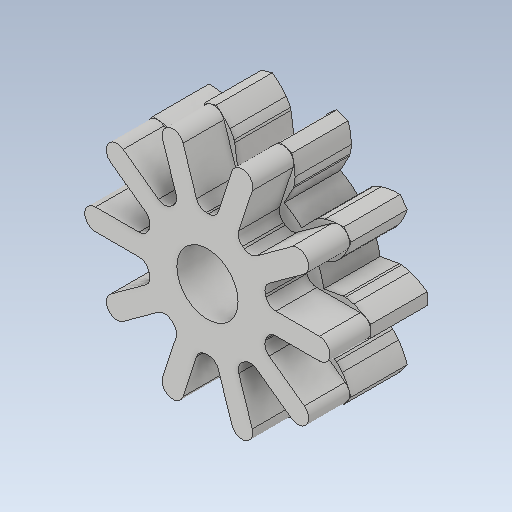
# Autodesk Inventor part: m2z10はめあい
Saved by Autodesk Inventor 2020 (Build 240168000, 168)
## iProperties
Created: 2019-05-28
Part Number: m2z10はめあい
Material: 一般
Document SubType Name: Modeling
Designer: hamaa
Density: 1 g/cm^3
Appearance: 既定
Mass: 2.32031 g
Surface Area: 20.1753 cm^2
Volume: 2.32031 cm^3
Author: hamaa
Autodesk Inventor part; units mm, degrees
ref_plane "YZ Plane" through (0, 0, 0) normal (1, 0, 0) x (0, 1, 0)
ref_plane "XZ Plane" through (0, 0, 0) normal (0, 1, 0) x (-1, 0, 0)
ref_plane "XY Plane" through (0, 0, 0) normal (0, 0, 1) x (1, 0, 0)
sketch "スケッチ1" plane through (0, 0, 0) normal (0, 0, 1) x (1, 0, 0)
  arc A0 (149.895, 114.5174) -> (149.8316, 114.302) centre (151.0075, 114.073) ccw
  arc A1 (150.3048, 115.256) -> (149.895, 114.5174) centre (153.0017, 113.2765) ccw
  arc A2 (151.645, 116.5804) -> (150.3048, 115.256) centre (155.1281, 111.7157) ccw
  arc A3 (144.0343, 113.5196) -> (144.1097, 113.3081) centre (145.1956, 113.8141) ccw
  arc A4 (143.9318, 114.3581) -> (144.0343, 113.5196) centre (147.2771, 114.3418) ccw
  arc A5 (144.2375, 116.2174) -> (143.9318, 114.3581) centre (149.9148, 114.329) ccw
  arc A6 (139.8794, 109.2677) -> (140.0647, 109.1408) centre (140.6459, 110.1884) ccw
  arc A7 (139.3036, 109.8857) -> (139.8794, 109.2677) centre (142.0196, 111.8388) ccw
  arc A8 (138.4581, 111.5696) -> (139.3036, 109.8857) centre (144.1611, 113.3789) ccw
  arc A9 (139.0173, 103.3856) -> (139.2417, 103.3918) centre (139.0961, 104.581) ccw
  arc A10 (138.1882, 103.5471) -> (139.0173, 103.3856) centre (139.2374, 106.7236) ccw
  arc A11 (136.5144, 104.4124) -> (138.1882, 103.5471) centre (140.0647, 109.2283) ccw
  arc A12 (141.7772, 98.1201) -> (141.9551, 98.2571) centre (141.1383, 99.1335) ccw
  arc A13 (141.0115, 97.7634) -> (141.7772, 98.1201) centre (139.9932, 100.95) ccw
  arc A14 (139.1487, 97.4797) -> (141.0115, 97.7634) centre (139.1903, 103.4626) ccw
  arc A15 (147.105, 95.4824) -> (147.1684, 95.6978) centre (145.9925, 95.9268) ccw
  arc A16 (146.6952, 94.7438) -> (147.105, 95.4824) centre (143.9983, 96.7233) ccw
  arc A17 (145.355, 93.4194) -> (146.6952, 94.7438) centre (141.8719, 98.2841) ccw
  arc A18 (152.9656, 96.4802) -> (152.8903, 96.6917) centre (151.8044, 96.1857) ccw
  arc A19 (153.0682, 95.6417) -> (152.9656, 96.4802) centre (149.7229, 95.658) ccw
  arc A20 (152.7625, 93.7824) -> (153.0682, 95.6417) centre (147.0852, 95.6708) ccw
  arc A21 (157.1206, 100.7321) -> (156.9353, 100.859) centre (156.3541, 99.8114) ccw
  arc A22 (157.6964, 100.1141) -> (157.1206, 100.7321) centre (154.9804, 98.161) ccw
  arc A23 (158.5419, 98.4302) -> (157.6964, 100.1141) centre (152.8389, 96.6209) ccw
  arc A24 (157.9827, 106.6143) -> (157.7583, 106.608) centre (157.9039, 105.4188) ccw
  arc A25 (158.8118, 106.4527) -> (157.9827, 106.6143) centre (157.7626, 103.2762) ccw
  arc A26 (160.4856, 105.5874) -> (158.8118, 106.4527) centre (156.9353, 100.7715) ccw
  arc A27 (155.2228, 111.8797) -> (155.0449, 111.7427) centre (155.8617, 110.8663) ccw
  arc A28 (155.9885, 112.2364) -> (155.2228, 111.8797) centre (157.0068, 109.0498) ccw
  arc A29 (157.8512, 112.5201) -> (155.9885, 112.2364) centre (157.8097, 106.5372) ccw
  arc A30 (147.1684, 114.302) -> (147.105, 114.5174) centre (145.9925, 114.073) ccw
  arc A31 (147.105, 114.5174) -> (146.6952, 115.256) centre (143.9983, 113.2765) ccw
  arc A32 (146.6952, 115.256) -> (145.355, 116.5804) centre (141.8719, 111.7157) ccw
  arc A33 (141.9551, 111.7427) -> (141.7772, 111.8797) centre (141.1383, 110.8663) ccw
  arc A34 (141.7772, 111.8797) -> (141.0115, 112.2364) centre (139.9932, 109.0498) ccw
  arc A35 (141.0115, 112.2364) -> (139.1487, 112.5201) centre (139.1903, 106.5372) ccw
  arc A36 (139.2417, 106.608) -> (139.0173, 106.6143) centre (139.0961, 105.4188) ccw
  arc A37 (139.0173, 106.6143) -> (138.1882, 106.4527) centre (139.2374, 103.2762) ccw
  arc A38 (138.1882, 106.4527) -> (136.5144, 105.5874) centre (140.0647, 100.7715) ccw
  arc A39 (140.0647, 100.859) -> (139.8794, 100.7321) centre (140.6459, 99.8114) ccw
  arc A40 (139.8794, 100.7321) -> (139.3036, 100.1141) centre (142.0196, 98.161) ccw
  arc A41 (139.3036, 100.1141) -> (138.4581, 98.4302) centre (144.1611, 96.6209) ccw
  arc A42 (144.1097, 96.6917) -> (144.0343, 96.4802) centre (145.1956, 96.1857) ccw
  arc A43 (144.0343, 96.4802) -> (143.9318, 95.6417) centre (147.2771, 95.658) ccw
  arc A44 (143.9318, 95.6417) -> (144.2375, 93.7824) centre (149.9148, 95.6708) ccw
  arc A45 (149.8316, 95.6978) -> (149.895, 95.4824) centre (151.0075, 95.9268) ccw
  arc A46 (149.895, 95.4824) -> (150.3048, 94.7438) centre (153.0017, 96.7233) ccw
  arc A47 (150.3048, 94.7438) -> (151.645, 93.4194) centre (155.1281, 98.2841) ccw
  arc A48 (155.0449, 98.2571) -> (155.2228, 98.1201) centre (155.8617, 99.1335) ccw
  arc A49 (155.2228, 98.1201) -> (155.9885, 97.7634) centre (157.0068, 100.95) ccw
  arc A50 (155.9885, 97.7634) -> (157.8512, 97.4797) centre (157.8097, 103.4626) ccw
  arc A51 (157.7583, 103.3918) -> (157.9827, 103.3856) centre (157.9039, 104.581) ccw
  arc A52 (157.9827, 103.3856) -> (158.8118, 103.5471) centre (157.7626, 106.7236) ccw
  arc A53 (158.8118, 103.5471) -> (160.4856, 104.4124) centre (156.9353, 109.2283) ccw
  arc A54 (156.9353, 109.1408) -> (157.1206, 109.2677) centre (156.3541, 110.1884) ccw
  arc A55 (157.1206, 109.2677) -> (157.6964, 109.8857) centre (154.9804, 111.8388) ccw
  arc A56 (157.6964, 109.8857) -> (158.5419, 111.5696) centre (152.8389, 113.3789) ccw
  arc A57 (152.8903, 113.3081) -> (152.9656, 113.5196) centre (151.8044, 113.8141) ccw
  arc A58 (152.9656, 113.5196) -> (153.0682, 114.3581) centre (149.7229, 114.3418) ccw
  arc A59 (153.0682, 114.3581) -> (152.7625, 116.2174) centre (147.0852, 114.329) ccw
  arc A60 (149.5628, 112.4242) -> (147.4372, 112.4242) centre (148.5, 104.9999) ccw
  arc A61 (144.9959, 111.631) -> (143.2763, 110.3816) centre (148.5, 104.9999) ccw
  arc A62 (141.7675, 108.3049) -> (141.1106, 106.2833) centre (148.5, 104.9999) ccw
  arc A63 (141.1106, 103.7165) -> (141.7675, 101.6949) centre (148.5, 104.9999) ccw
  arc A64 (143.2763, 99.6182) -> (144.9959, 98.3688) centre (148.5, 104.9999) ccw
  arc A65 (147.4372, 97.5756) -> (149.5628, 97.5756) centre (148.5, 104.9999) ccw
  arc A66 (152.0041, 98.3688) -> (153.7237, 99.6182) centre (148.5, 104.9999) ccw
  arc A67 (155.2325, 101.6949) -> (155.8894, 103.7165) centre (148.5, 104.9999) ccw
  arc A68 (155.8894, 106.2833) -> (155.2325, 108.3049) centre (148.5, 104.9999) ccw
  arc A69 (153.7237, 110.3816) -> (152.0041, 111.631) centre (148.5, 104.9999) ccw
  arc A70 (145.355, 116.5804) -> (144.2375, 116.2174) centre (148.5, 104.9999) ccw
  arc A71 (139.1487, 112.5201) -> (138.4581, 111.5696) centre (148.5, 104.9999) ccw
  arc A72 (136.5144, 105.5874) -> (136.5144, 104.4124) centre (148.5, 104.9999) ccw
  arc A73 (138.4581, 98.4302) -> (139.1487, 97.4797) centre (148.5, 104.9999) ccw
  arc A74 (144.2375, 93.7824) -> (145.355, 93.4194) centre (148.5, 104.9999) ccw
  arc A75 (151.645, 93.4194) -> (152.7625, 93.7824) centre (148.5, 104.9999) ccw
  arc A76 (157.8512, 97.4797) -> (158.5419, 98.4302) centre (148.5, 104.9999) ccw
  arc A77 (160.4856, 104.4124) -> (160.4856, 105.5874) centre (148.5, 104.9999) ccw
  arc A78 (158.5419, 111.5696) -> (157.8512, 112.5201) centre (148.5, 104.9999) ccw
  arc A79 (152.7625, 116.2174) -> (151.645, 116.5804) centre (148.5, 104.9999) ccw
  line L0 (149.5628, 112.4242) -> (149.8316, 114.302)
  line L1 (144.9959, 111.631) -> (144.1097, 113.3081)
  line L2 (141.7675, 108.3049) -> (140.0647, 109.1408)
  line L3 (141.1106, 103.7165) -> (139.2417, 103.3918)
  line L4 (143.2763, 99.6182) -> (141.9551, 98.2571)
  line L5 (147.4372, 97.5756) -> (147.1684, 95.6978)
  line L6 (152.0041, 98.3688) -> (152.8903, 96.6917)
  line L7 (155.2325, 101.6949) -> (156.9353, 100.859)
  line L8 (155.8894, 106.2833) -> (157.7583, 106.608)
  line L9 (153.7237, 110.3816) -> (155.0449, 111.7427)
  line L10 (147.4372, 112.4242) -> (147.1684, 114.302)
  line L11 (143.2763, 110.3816) -> (141.9551, 111.7427)
  line L12 (141.1106, 106.2833) -> (139.2417, 106.608)
  line L13 (141.7675, 101.6949) -> (140.0647, 100.859)
  line L14 (144.9959, 98.3688) -> (144.1097, 96.6917)
  line L15 (149.5628, 97.5756) -> (149.8316, 95.6978)
  line L16 (153.7237, 99.6182) -> (155.0449, 98.2571)
  line L17 (155.8894, 103.7165) -> (157.7583, 103.3918)
  line L18 (155.2325, 108.3049) -> (156.9353, 109.1408)
  line L19 (152.0041, 111.631) -> (152.8903, 113.3081)
  line L20 (134.5, 105) -> (162.5, 105)
  line L21 (148.5, 91) -> (148.5, 119)
  line L22 (180.5, 116.9999) -> (250.5, 116.9999)
  line L23 (180.5, 108.9999) -> (250.5, 108.9999)
  line L24 (180.5, 100.9999) -> (250.5, 100.9999)
  line L25 (180.5, 92.9999) -> (250.5, 92.9999)
  line L26 (180.5, 84.9999) -> (250.5, 84.9999)
  line L27 (180.5, 76.9999) -> (250.5, 76.9999)
  line L28 (180.5, 68.9999) -> (250.5, 68.9999)
  line L29 (180.5, 60.9999) -> (250.5, 60.9999)
  line L30 (180.5, 52.9999) -> (250.5, 52.9999)
  line L31 (180.5, 44.9999) -> (250.5, 44.9999)
  line L32 (180.5, 36.9999) -> (250.5, 36.9999)
  line L33 (180.5, 28.9999) -> (250.5, 28.9999)
  line L34 (180.5, 20.9999) -> (250.5, 20.9999)
  line L35 (180.5, 116.9999) -> (180.5, 20.9999)
  line L36 (250.5, 116.9999) -> (250.5, 20.9999)
  line L37 (215.5, 108.9999) -> (215.5, 20.9999)
  point P0 (0, 0)
  point P1 (186.5, 111)
  point P2 (189, 103)
  point P3 (189, 95)
  point P4 (186.5, 87)
  point P5 (189, 79)
  point P6 (184, 71)
  point P7 (186.5, 63)
  point P8 (186.5, 55)
  point P9 (186.5, 47)
  point P10 (189, 39)
  point P11 (189, 31)
  point P12 (186.5, 23)
  point P13 (216.5, 103)
  point P14 (231.5, 95)
  point P15 (232.75, 87)
  point P16 (229, 79)
  point P17 (231.5, 71)
  point P18 (225.25, 63)
  point P19 (231.5, 55)
  point P20 (231.5, 47)
  point P21 (226.5, 39)
  point P22 (234, 31)
  point P23 (234, 23)
  point P24 (149.5, 132.5)
  point P25 (149.5, 126.5)
  point P26 (166.75, 132.5)
  point P27 (167.8125, 126.5)
  constraints: 160 point on circle, 80 centre point, 72 end point, 60 tangent, 57 equal radius, 23 parallel, 2 horizontal, 2 midpoint, 2 perpendicular, 55 other
extrude "押し出し1" add sketch "スケッチ1" along normal blind 5.5 contours A1 A2 A79 A59 A58 A57 L19 A69 L9 A27 A28 A29 A78 A56 A55 A54 L18 A68 L8 A24 A25 A26 A77 L20 L21 A60 L0 A0 | L21 L20 A72 A38 A37 A36 L12 A62 L2 A6 A7 A8 A71 A35 A34 A33 L11 A61 L1 A3 A4 A5 A70 A32 A31 A30 L10 A60 | L21 A65 L5 A15 A16 A17 A74 A44 A43 A42 L14 A64 L4 A12 A13 A14 A73 A41 A40 A39 L13 A63 L3 A9 A10 A11 A72 L20 | L20 A77 A53 A52 A51 L17 A67 L7 A21 A22 A23 A76 A50 A49 A48 L16 A66 L6 A18 A19 A20 A75 A47 A46 A45 L15 A65 L21
sketch "スケッチ3" plane through (0, 0, 5.5) normal (0, 0, 1) x (1, 0, 0)
  arc A0 (149.895, 114.5174) -> (149.8316, 114.302) centre (151.0075, 114.073) ccw projected
  line L0 (149.8316, 114.302) -> (149.5628, 112.4242) projected
  arc A1 (149.5628, 112.4242) -> (147.4372, 112.4242) centre (148.5, 104.9999) ccw projected
  line L1 (147.4372, 112.4242) -> (147.1684, 114.302) projected
  arc A2 (147.1684, 114.302) -> (147.105, 114.5174) centre (145.9925, 114.073) ccw projected
  arc A3 (147.105, 114.5174) -> (146.6952, 115.256) centre (143.9983, 113.2765) ccw projected
  arc A4 (146.6952, 115.256) -> (145.355, 116.5804) centre (141.8719, 111.7157) ccw projected
  arc A5 (145.355, 116.5804) -> (144.2375, 116.2174) centre (148.5, 104.9999) ccw projected
  arc A6 (144.2375, 116.2174) -> (143.9318, 114.3581) centre (149.9148, 114.329) ccw projected
  arc A7 (143.9318, 114.3581) -> (144.0343, 113.5196) centre (147.2771, 114.3418) ccw projected
  arc A8 (144.0343, 113.5196) -> (144.1097, 113.3081) centre (145.1956, 113.8141) ccw projected
  line L2 (144.1097, 113.3081) -> (144.9959, 111.631) projected
  arc A9 (144.9959, 111.631) -> (143.2763, 110.3816) centre (148.5, 104.9999) ccw projected
  line L3 (143.2763, 110.3816) -> (141.9551, 111.7427) projected
  arc A10 (141.9551, 111.7427) -> (141.7772, 111.8797) centre (141.1383, 110.8663) ccw projected
  arc A11 (141.7772, 111.8797) -> (141.0115, 112.2364) centre (139.9932, 109.0498) ccw projected
  arc A12 (141.0115, 112.2364) -> (139.1487, 112.5201) centre (139.1903, 106.5372) ccw projected
  arc A13 (139.1487, 112.5201) -> (138.4581, 111.5696) centre (148.5, 104.9999) ccw projected
  arc A14 (138.4581, 111.5696) -> (139.3036, 109.8857) centre (144.1611, 113.3789) ccw projected
  arc A15 (139.3036, 109.8857) -> (139.8794, 109.2677) centre (142.0196, 111.8388) ccw projected
  arc A16 (139.8794, 109.2677) -> (140.0647, 109.1408) centre (140.6459, 110.1884) ccw projected
  line L4 (140.0647, 109.1408) -> (141.7675, 108.3049) projected
  arc A17 (141.7675, 108.3049) -> (141.1106, 106.2833) centre (148.5, 104.9999) ccw projected
  line L5 (141.1106, 106.2833) -> (139.2417, 106.608) projected
  arc A18 (139.2417, 106.608) -> (139.0173, 106.6143) centre (139.0961, 105.4188) ccw projected
  arc A19 (139.0173, 106.6143) -> (138.1882, 106.4527) centre (139.2374, 103.2762) ccw projected
  arc A20 (138.1882, 106.4527) -> (136.5144, 105.5874) centre (140.0647, 100.7715) ccw projected
  arc A21 (136.5144, 105.5874) -> (136.5144, 104.4124) centre (148.5, 104.9999) ccw projected
  arc A22 (136.5144, 104.4124) -> (138.1882, 103.5471) centre (140.0647, 109.2283) ccw projected
  arc A23 (138.1882, 103.5471) -> (139.0173, 103.3856) centre (139.2374, 106.7236) ccw projected
  arc A24 (139.0173, 103.3856) -> (139.2417, 103.3918) centre (139.0961, 104.581) ccw projected
  line L6 (139.2417, 103.3918) -> (141.1106, 103.7165) projected
  arc A25 (141.1106, 103.7165) -> (141.7675, 101.6949) centre (148.5, 104.9999) ccw projected
  line L7 (141.7675, 101.6949) -> (140.0647, 100.859) projected
  arc A26 (140.0647, 100.859) -> (139.8794, 100.7321) centre (140.6459, 99.8114) ccw projected
  arc A27 (139.8794, 100.7321) -> (139.3036, 100.1141) centre (142.0196, 98.161) ccw projected
  arc A28 (139.3036, 100.1141) -> (138.4581, 98.4302) centre (144.1611, 96.6209) ccw projected
  arc A29 (138.4581, 98.4302) -> (139.1487, 97.4797) centre (148.5, 104.9999) ccw projected
  arc A30 (139.1487, 97.4797) -> (141.0115, 97.7634) centre (139.1903, 103.4626) ccw projected
  arc A31 (141.0115, 97.7634) -> (141.7772, 98.1201) centre (139.9932, 100.95) ccw projected
  arc A32 (141.7772, 98.1201) -> (141.9551, 98.2571) centre (141.1383, 99.1335) ccw projected
  line L8 (141.9551, 98.2571) -> (143.2763, 99.6182) projected
  arc A33 (143.2763, 99.6182) -> (144.9959, 98.3688) centre (148.5, 104.9999) ccw projected
  line L9 (144.9959, 98.3688) -> (144.1097, 96.6917) projected
  arc A34 (144.1097, 96.6917) -> (144.0343, 96.4802) centre (145.1956, 96.1857) ccw projected
  arc A35 (144.0343, 96.4802) -> (143.9318, 95.6417) centre (147.2771, 95.658) ccw projected
  arc A36 (143.9318, 95.6417) -> (144.2375, 93.7824) centre (149.9148, 95.6708) ccw projected
  arc A37 (144.2375, 93.7824) -> (145.355, 93.4194) centre (148.5, 104.9999) ccw projected
  arc A38 (145.355, 93.4194) -> (146.6952, 94.7438) centre (141.8719, 98.2841) ccw projected
  arc A39 (146.6952, 94.7438) -> (147.105, 95.4824) centre (143.9983, 96.7233) ccw projected
  arc A40 (147.105, 95.4824) -> (147.1684, 95.6978) centre (145.9925, 95.9268) ccw projected
  line L10 (147.1684, 95.6978) -> (147.4372, 97.5756) projected
  arc A41 (147.4372, 97.5756) -> (149.5628, 97.5756) centre (148.5, 104.9999) ccw projected
  line L11 (149.5628, 97.5756) -> (149.8316, 95.6978) projected
  arc A42 (149.8316, 95.6978) -> (149.895, 95.4824) centre (151.0075, 95.9268) ccw projected
  arc A43 (149.895, 95.4824) -> (150.3048, 94.7438) centre (153.0017, 96.7233) ccw projected
  arc A44 (150.3048, 94.7438) -> (151.645, 93.4194) centre (155.1281, 98.2841) ccw projected
  arc A45 (151.645, 93.4194) -> (152.7625, 93.7824) centre (148.5, 104.9999) ccw projected
  arc A46 (152.7625, 93.7824) -> (153.0682, 95.6417) centre (147.0852, 95.6708) ccw projected
  arc A47 (153.0682, 95.6417) -> (152.9656, 96.4802) centre (149.7229, 95.658) ccw projected
  arc A48 (152.9656, 96.4802) -> (152.8903, 96.6917) centre (151.8044, 96.1857) ccw projected
  line L12 (152.8903, 96.6917) -> (152.0041, 98.3688) projected
  arc A49 (152.0041, 98.3688) -> (153.7237, 99.6182) centre (148.5, 104.9999) ccw projected
  line L13 (153.7237, 99.6182) -> (155.0449, 98.2571) projected
  arc A50 (155.0449, 98.2571) -> (155.2228, 98.1201) centre (155.8617, 99.1335) ccw projected
  arc A51 (155.2228, 98.1201) -> (155.9885, 97.7634) centre (157.0068, 100.95) ccw projected
  arc A52 (155.9885, 97.7634) -> (157.8512, 97.4797) centre (157.8097, 103.4626) ccw projected
  arc A53 (157.8512, 97.4797) -> (158.5419, 98.4302) centre (148.5, 104.9999) ccw projected
  arc A54 (158.5419, 98.4302) -> (157.6964, 100.1141) centre (152.8389, 96.6209) ccw projected
  arc A55 (157.6964, 100.1141) -> (157.1206, 100.7321) centre (154.9804, 98.161) ccw projected
  arc A56 (157.1206, 100.7321) -> (156.9353, 100.859) centre (156.3541, 99.8114) ccw projected
  line L14 (156.9353, 100.859) -> (155.2325, 101.6949) projected
  arc A57 (155.2325, 101.6949) -> (155.8894, 103.7165) centre (148.5, 104.9999) ccw projected
  line L15 (155.8894, 103.7165) -> (157.7583, 103.3918) projected
  arc A58 (157.7583, 103.3918) -> (157.9827, 103.3856) centre (157.9039, 104.581) ccw projected
  arc A59 (157.9827, 103.3856) -> (158.8118, 103.5471) centre (157.7626, 106.7236) ccw projected
  arc A60 (158.8118, 103.5471) -> (160.4856, 104.4124) centre (156.9353, 109.2283) ccw projected
  arc A61 (160.4856, 104.4124) -> (160.4856, 105.5874) centre (148.5, 104.9999) ccw projected
  arc A62 (160.4856, 105.5874) -> (158.8118, 106.4527) centre (156.9353, 100.7715) ccw projected
  arc A63 (158.8118, 106.4527) -> (157.9827, 106.6143) centre (157.7626, 103.2762) ccw projected
  arc A64 (157.9827, 106.6143) -> (157.7583, 106.608) centre (157.9039, 105.4188) ccw projected
  line L16 (157.7583, 106.608) -> (155.8894, 106.2833) projected
  arc A65 (155.8894, 106.2833) -> (155.2325, 108.3049) centre (148.5, 104.9999) ccw projected
  line L17 (155.2325, 108.3049) -> (156.9353, 109.1408) projected
  arc A66 (156.9353, 109.1408) -> (157.1206, 109.2677) centre (156.3541, 110.1884) ccw projected
  arc A67 (157.1206, 109.2677) -> (157.6964, 109.8857) centre (154.9804, 111.8388) ccw projected
  arc A68 (157.6964, 109.8857) -> (158.5419, 111.5696) centre (152.8389, 113.3789) ccw projected
  arc A69 (158.5419, 111.5696) -> (157.8512, 112.5201) centre (148.5, 104.9999) ccw projected
  arc A70 (157.8512, 112.5201) -> (155.9885, 112.2364) centre (157.8097, 106.5372) ccw projected
  arc A71 (155.9885, 112.2364) -> (155.2228, 111.8797) centre (157.0068, 109.0498) ccw projected
  arc A72 (155.2228, 111.8797) -> (155.0449, 111.7427) centre (155.8617, 110.8663) ccw projected
  line L18 (155.0449, 111.7427) -> (153.7237, 110.3816) projected
  arc A73 (153.7237, 110.3816) -> (152.0041, 111.631) centre (148.5, 104.9999) ccw projected
  line L19 (152.0041, 111.631) -> (152.8903, 113.3081) projected
  arc A74 (152.8903, 113.3081) -> (152.9656, 113.5196) centre (151.8044, 113.8141) ccw projected
  arc A75 (152.9656, 113.5196) -> (153.0682, 114.3581) centre (149.7229, 114.3418) ccw projected
  arc A76 (153.0682, 114.3581) -> (152.7625, 116.2174) centre (147.0852, 114.329) ccw projected
  arc A77 (152.7625, 116.2174) -> (151.645, 116.5804) centre (148.5, 104.9999) ccw projected
  arc A78 (151.645, 116.5804) -> (150.3048, 115.256) centre (155.1281, 111.7157) ccw projected
  arc A79 (150.3048, 115.256) -> (149.895, 114.5174) centre (153.0017, 113.2765) ccw projected
  line L20 (145.1163, 115.414) -> (151.8837, 94.5858) construction
  line L21 (144.1176, 115.0895) -> (150.8851, 94.2614)
  line L22 (152.8823, 94.9103) -> (146.1149, 115.7384)
  arc A80 (146.1149, 115.7384) -> (144.1176, 115.0895) centre (145.1163, 115.414) ccw
  arc A81 (150.8851, 94.2614) -> (152.8823, 94.9103) centre (151.8837, 94.5858) ccw
  line L23 (157.3587, 111.4362) -> (159.45, 104.9999) construction
  line L24 (159.45, 104.9999) -> (157.3587, 98.5637) construction
  line L25 (157.3587, 98.5637) -> (151.8837, 94.5858) construction
  line L26 (151.8837, 94.5858) -> (145.1163, 94.5858) construction
  line L27 (145.1163, 94.5858) -> (139.6413, 98.5637) construction
  line L28 (139.6413, 98.5637) -> (137.55, 104.9999) construction
  line L29 (137.55, 104.9999) -> (139.6413, 111.4362) construction
  line L30 (139.6413, 111.4362) -> (145.1163, 115.414) construction
  line L31 (145.1163, 115.414) -> (151.8837, 115.414) construction
  line L32 (151.8837, 115.414) -> (157.3587, 111.4362) construction
  arc A82 (145.355, 116.5804) -> (144.2375, 116.2174) centre (148.5, 104.9999) ccw projected
  line L33 (139.6413, 111.4362) -> (157.3587, 98.5637) construction
  line L34 (139.0241, 110.5867) -> (156.7416, 97.7142)
  line L35 (157.9759, 99.4131) -> (140.2584, 112.2856)
  arc A83 (140.2584, 112.2856) -> (139.0241, 110.5867) centre (139.6413, 111.4362) ccw
  arc A84 (156.7416, 97.7142) -> (157.9759, 99.4131) centre (157.3587, 98.5637) ccw
  line L36 (151.8837, 115.414) -> (145.1163, 94.5858) construction
  line L37 (150.8851, 115.7384) -> (144.1176, 94.9103)
  line L38 (146.1149, 94.2614) -> (152.8823, 115.0895)
  arc A85 (152.8823, 115.0895) -> (150.8851, 115.7384) centre (151.8837, 115.414) ccw
  arc A86 (144.1176, 94.9103) -> (146.1149, 94.2614) centre (145.1163, 94.5858) ccw
  line L39 (159.45, 104.9999) -> (137.55, 104.9999) construction
  line L40 (159.45, 106.0499) -> (137.55, 106.0499)
  line L41 (137.55, 103.9499) -> (159.45, 103.9499)
  arc A87 (159.45, 103.9499) -> (159.45, 106.0499) centre (159.45, 104.9999) ccw
  arc A88 (137.55, 106.0499) -> (137.55, 103.9499) centre (137.55, 104.9999) ccw
  line L42 (157.3587, 111.4362) -> (139.6413, 98.5637) construction
  line L43 (156.7416, 112.2856) -> (139.0241, 99.4131)
  line L44 (140.2584, 97.7142) -> (157.9759, 110.5867)
  arc A89 (157.9759, 110.5867) -> (156.7416, 112.2856) centre (157.3587, 111.4362) ccw
  arc A90 (139.0241, 99.4131) -> (140.2584, 97.7142) centre (139.6413, 98.5637) ccw
  circle A91 centre (148.5, 104.9999) radius 6
  point P0 (0, 0)
  point P1 (148.5, 104.9999)
  point P2 (148.5, 104.9999)
  point P3 (148.5, 104.9999)
  dimension "d8" = 2.1
  dimension "d9" = 2.1
  dimension "d10" = 2.1
  dimension "d11" = 2.1
  dimension "d12" = 2.1
  dimension "d13" = 12
  constraints: 60 end point, 21 tangent, 20 point on circle, 11 centre point, 5 midpoint, 5 parallel, 3 coincident, 2 horizontal, 21 other
  measures "d8" diameter of A81
  measures "d9" diameter of A84
  measures "d10" diameter of A86
  measures "d11" diameter of A88
  measures "d12" diameter of A90
  measures "d13" diameter of A91
extrude "押し出し4" add sketch "スケッチ3" along normal blind 4 contours A85 L38 A91 L37 | A91 L43 L38 | L38 L43 L22 L37 A91 | L37 L22 A91 | L43 A91 L44 L40 L38 | L38 L40 L22 L43 | L43 A89 L44 A91 | L37 L35 L21 A91 L22 | L22 L43 L35 L37 | A91 L21 A80 L22 | L40 L44 L35 L38 | L38 L35 L22 L40 | L22 L40 L35 L43 | A91 L40 L44 | L37 L40 L21 L35 | L35 L43 L40 L37 | L21 L35 A91 | L38 L22 L35 | L35 L44 L22 L38 | L40 A91 L41 L35 L44 | L22 L35 L40 | L35 L40 L43 | L40 A87 L41 A91 | L21 L40 L34 A91 L35 | L40 L43 L37 | L37 L43 L21 L40 | A91 L34 A83 L35 | L35 L41 L22 L44 | L22 L38 L44 L41 L34 L21 L37 L43 L40 L35 | L22 L44 L38 | L21 L43 L34 L40 | L37 L21 L43 | L34 L40 A91 | L41 A91 L35 | L35 A91 L34 L22 L41 | L22 L41 L38 L44 | L38 L41 L44 | L21 L37 L34 L43 | L34 L43 L41 A91 L40 | L21 L34 L37 | A91 L41 A88 L40 | L35 A84 L34 A91 | L22 L34 L38 L41 | L38 L34 L44 L41 | L44 L34 L41 | L34 L37 L41 L43 | L34 L41 L21 | L21 L41 L37 L34 | L41 L43 A91 | A91 L22 L34 | L22 A91 L21 L38 L34 | L38 L21 L44 L34 | L34 L44 L21 L41 | L41 L37 L44 A91 L43 | L21 L44 L37 L41 | A91 L44 A90 L43 | L22 A81 L21 A91 | L38 A91 L37 L44 L21 | L21 A91 L38 | L37 A91 L44 | L38 A86 L37 A91
fillet "フィレット1" radius 1 20 edges at (147.6731, 110.9427, 7.5) (151.3241, 99.7061, 7.5) (145.6759, 110.2937, 7.5) (149.3269, 99.0572, 7.5) (153.8964, 102.3771, 7.5) (144.338, 109.3217, 7.5) (151.3241, 110.2937, 7.5) (147.6731, 99.0572, 7.5) (149.3269, 110.9427, 7.5) (145.6759, 99.7061, 7.5) (152.662, 109.3217, 7.5) (143.1036, 102.3771, 7.5) (153.8964, 107.6227, 7.5) (144.338, 100.6781, 7.5) (154.4074, 106.0499, 7.5) (142.5926, 106.0499, 7.5) (154.4074, 103.9499, 7.5) (142.5926, 103.9499, 7.5) (152.662, 100.6781, 7.5) (143.1036, 107.6227, 7.5)
sketch "スケッチ4" plane through (0, 0, 9.5) normal (0, 0, 1) x (1, 0, 0)
  arc A0 (154.1741, 103.0494) -> (154.2369, 103.2428) centre (148.5, 104.9999) ccw projected
  arc A1 (155.1931, 103.9499) -> (154.2369, 103.2428) centre (155.1931, 102.9499) ccw projected
  line L0 (155.1931, 103.9499) -> (159.45, 103.9499) projected
  arc A2 (159.45, 103.9499) -> (159.45, 106.0499) centre (159.45, 104.9999) ccw projected
  line L1 (159.45, 106.0499) -> (155.1931, 106.0499) projected
  arc A3 (154.2369, 106.757) -> (155.1931, 106.0499) centre (155.1931, 107.0499) ccw projected
  arc A4 (154.2369, 106.757) -> (154.1741, 106.9504) centre (148.5, 104.9999) ccw projected
  arc A5 (154.532, 108.0845) -> (154.1741, 106.9504) centre (155.1198, 107.2755) ccw projected
  line L2 (154.532, 108.0845) -> (157.9759, 110.5867) projected
  arc A6 (157.9759, 110.5867) -> (156.7416, 112.2856) centre (157.3587, 111.4362) ccw projected
  line L3 (156.7416, 112.2856) -> (153.2976, 109.7835) projected
  arc A7 (152.1084, 109.7935) -> (153.2976, 109.7835) centre (152.7099, 110.5925) ccw projected
  arc A8 (152.1084, 109.7935) -> (151.9439, 109.9131) centre (148.5, 104.9999) ccw projected
  arc A9 (151.5669, 111.0409) -> (151.9439, 109.9131) centre (152.5179, 110.7319) ccw projected
  line L4 (151.5669, 111.0409) -> (152.8823, 115.0895) projected
  arc A10 (152.8823, 115.0895) -> (150.8851, 115.7384) centre (151.8837, 115.414) ccw projected
  line L5 (150.8851, 115.7384) -> (149.5697, 111.6899) projected
  arc A11 (148.6017, 110.999) -> (149.5697, 111.6899) centre (148.6186, 111.9989) ccw projected
  arc A12 (148.6017, 110.999) -> (148.3983, 110.999) centre (148.5, 104.9999) ccw projected
  arc A13 (147.4303, 111.6899) -> (148.3983, 110.999) centre (148.3814, 111.9989) ccw projected
  line L6 (147.4303, 111.6899) -> (146.1149, 115.7384) projected
  arc A14 (146.1149, 115.7384) -> (144.1176, 115.0895) centre (145.1163, 115.414) ccw projected
  line L7 (144.1176, 115.0895) -> (145.4331, 111.0409) projected
  arc A15 (145.056, 109.9131) -> (145.4331, 111.0409) centre (144.482, 110.7319) ccw projected
  arc A16 (145.056, 109.9131) -> (144.8915, 109.7935) centre (148.5, 104.9999) ccw projected
  arc A17 (143.7023, 109.7835) -> (144.8915, 109.7935) centre (144.2901, 110.5925) ccw projected
  line L8 (143.7023, 109.7835) -> (140.2584, 112.2856) projected
  arc A18 (140.2584, 112.2856) -> (139.0241, 110.5867) centre (139.6413, 111.4362) ccw projected
  line L9 (139.0241, 110.5867) -> (142.468, 108.0845) projected
  arc A19 (142.8259, 106.9504) -> (142.468, 108.0845) centre (141.8802, 107.2755) ccw projected
  arc A20 (142.8259, 106.9504) -> (142.7631, 106.757) centre (148.5, 104.9999) ccw projected
  arc A21 (141.8069, 106.0499) -> (142.7631, 106.757) centre (141.8069, 107.0499) ccw projected
  line L10 (141.8069, 106.0499) -> (137.55, 106.0499) projected
  arc A22 (137.55, 106.0499) -> (137.55, 103.9499) centre (137.55, 104.9999) ccw projected
  line L11 (137.55, 103.9499) -> (141.8069, 103.9499) projected
  arc A23 (142.7631, 103.2428) -> (141.8069, 103.9499) centre (141.8069, 102.9499) ccw projected
  arc A24 (142.7631, 103.2428) -> (142.8259, 103.0494) centre (148.5, 104.9999) ccw projected
  arc A25 (142.468, 101.9153) -> (142.8259, 103.0494) centre (141.8802, 102.7243) ccw projected
  line L12 (142.468, 101.9153) -> (139.0241, 99.4131) projected
  arc A26 (139.0241, 99.4131) -> (140.2584, 97.7142) centre (139.6413, 98.5637) ccw projected
  line L13 (140.2584, 97.7142) -> (143.7023, 100.2163) projected
  arc A27 (144.8915, 100.2063) -> (143.7023, 100.2163) centre (144.2901, 99.4073) ccw projected
  arc A28 (144.8915, 100.2063) -> (145.056, 100.0867) centre (148.5, 104.9999) ccw projected
  arc A29 (145.4331, 98.9589) -> (145.056, 100.0867) centre (144.482, 99.2679) ccw projected
  line L14 (145.4331, 98.9589) -> (144.1176, 94.9103) projected
  arc A30 (144.1176, 94.9103) -> (146.1149, 94.2614) centre (145.1163, 94.5858) ccw projected
  line L15 (146.1149, 94.2614) -> (147.4303, 98.3099) projected
  arc A31 (148.3983, 99.0008) -> (147.4303, 98.3099) centre (148.3814, 98.0009) ccw projected
  arc A32 (148.3983, 99.0008) -> (148.6017, 99.0008) centre (148.5, 104.9999) ccw projected
  arc A33 (149.5697, 98.3099) -> (148.6017, 99.0008) centre (148.6186, 98.0009) ccw projected
  line L16 (149.5697, 98.3099) -> (150.8851, 94.2614) projected
  arc A34 (150.8851, 94.2614) -> (152.8823, 94.9103) centre (151.8837, 94.5858) ccw projected
  line L17 (152.8823, 94.9103) -> (151.5669, 98.9589) projected
  arc A35 (151.9439, 100.0867) -> (151.5669, 98.9589) centre (152.5179, 99.2679) ccw projected
  arc A36 (151.9439, 100.0867) -> (152.1084, 100.2063) centre (148.5, 104.9999) ccw projected
  arc A37 (153.2976, 100.2163) -> (152.1084, 100.2063) centre (152.7099, 99.4073) ccw projected
  line L18 (153.2976, 100.2163) -> (156.7416, 97.7142) projected
  arc A38 (156.7416, 97.7142) -> (157.9759, 99.4131) centre (157.3587, 98.5637) ccw projected
  line L19 (157.9759, 99.4131) -> (154.532, 101.9153) projected
  arc A39 (154.1741, 103.0494) -> (154.532, 101.9153) centre (155.1198, 102.7243) ccw projected
  circle A40 centre (148.5, 104.9999) radius 2.995
  point P0 (0, 0)
  dimension "d17" = 5.99
  constraints: 1 centre point, 1 coincident
  measures "d17" diameter of A40
extrude "押し出し5" cut sketch "スケッチ4" against normal blind 10 contours A40
sketch "スケッチ6" plane through (0, 0, 9.5) normal (0, 0, 1) x (1, 0, 0)
  circle A0 centre (148.5, 104.9999) radius 2.995 projected
  arc A1 (154.1741, 103.0494) -> (154.2369, 103.2428) centre (148.5, 104.9999) ccw projected
  arc A2 (155.1931, 103.9499) -> (154.2369, 103.2428) centre (155.1931, 102.9499) ccw projected
  line L0 (155.1931, 103.9499) -> (159.45, 103.9499) projected
  arc A3 (159.45, 103.9499) -> (159.45, 106.0499) centre (159.45, 104.9999) ccw projected
  line L1 (159.45, 106.0499) -> (155.1931, 106.0499) projected
  arc A4 (154.2369, 106.757) -> (155.1931, 106.0499) centre (155.1931, 107.0499) ccw projected
  arc A5 (154.2369, 106.757) -> (154.1741, 106.9504) centre (148.5, 104.9999) ccw projected
  arc A6 (154.532, 108.0845) -> (154.1741, 106.9504) centre (155.1198, 107.2755) ccw projected
  line L2 (154.532, 108.0845) -> (157.9759, 110.5867) projected
  arc A7 (157.9759, 110.5867) -> (156.7416, 112.2856) centre (157.3587, 111.4362) ccw projected
  line L3 (156.7416, 112.2856) -> (153.2976, 109.7835) projected
  arc A8 (152.1084, 109.7935) -> (153.2976, 109.7835) centre (152.7099, 110.5925) ccw projected
  arc A9 (152.1084, 109.7935) -> (151.9439, 109.9131) centre (148.5, 104.9999) ccw projected
  arc A10 (151.5669, 111.0409) -> (151.9439, 109.9131) centre (152.5179, 110.7319) ccw projected
  line L4 (151.5669, 111.0409) -> (152.8823, 115.0895) projected
  arc A11 (152.8823, 115.0895) -> (150.8851, 115.7384) centre (151.8837, 115.414) ccw projected
  line L5 (150.8851, 115.7384) -> (149.5697, 111.6899) projected
  arc A12 (148.6017, 110.999) -> (149.5697, 111.6899) centre (148.6186, 111.9989) ccw projected
  arc A13 (148.6017, 110.999) -> (148.3983, 110.999) centre (148.5, 104.9999) ccw projected
  arc A14 (147.4303, 111.6899) -> (148.3983, 110.999) centre (148.3814, 111.9989) ccw projected
  line L6 (147.4303, 111.6899) -> (146.1149, 115.7384) projected
  arc A15 (146.1149, 115.7384) -> (144.1176, 115.0895) centre (145.1163, 115.414) ccw projected
  line L7 (144.1176, 115.0895) -> (145.4331, 111.0409) projected
  arc A16 (145.056, 109.9131) -> (145.4331, 111.0409) centre (144.482, 110.7319) ccw projected
  arc A17 (145.056, 109.9131) -> (144.8915, 109.7935) centre (148.5, 104.9999) ccw projected
  arc A18 (143.7023, 109.7835) -> (144.8915, 109.7935) centre (144.2901, 110.5925) ccw projected
  line L8 (143.7023, 109.7835) -> (140.2584, 112.2856) projected
  arc A19 (140.2584, 112.2856) -> (139.0241, 110.5867) centre (139.6413, 111.4362) ccw projected
  line L9 (139.0241, 110.5867) -> (142.468, 108.0845) projected
  arc A20 (142.8259, 106.9504) -> (142.468, 108.0845) centre (141.8802, 107.2755) ccw projected
  arc A21 (142.8259, 106.9504) -> (142.7631, 106.757) centre (148.5, 104.9999) ccw projected
  arc A22 (141.8069, 106.0499) -> (142.7631, 106.757) centre (141.8069, 107.0499) ccw projected
  line L10 (141.8069, 106.0499) -> (137.55, 106.0499) projected
  arc A23 (137.55, 106.0499) -> (137.55, 103.9499) centre (137.55, 104.9999) ccw projected
  line L11 (137.55, 103.9499) -> (141.8069, 103.9499) projected
  arc A24 (142.7631, 103.2428) -> (141.8069, 103.9499) centre (141.8069, 102.9499) ccw projected
  arc A25 (142.7631, 103.2428) -> (142.8259, 103.0494) centre (148.5, 104.9999) ccw projected
  arc A26 (142.468, 101.9153) -> (142.8259, 103.0494) centre (141.8802, 102.7243) ccw projected
  line L12 (142.468, 101.9153) -> (139.0241, 99.4131) projected
  arc A27 (139.0241, 99.4131) -> (140.2584, 97.7142) centre (139.6413, 98.5637) ccw projected
  line L13 (140.2584, 97.7142) -> (143.7023, 100.2163) projected
  arc A28 (144.8915, 100.2063) -> (143.7023, 100.2163) centre (144.2901, 99.4073) ccw projected
  arc A29 (144.8915, 100.2063) -> (145.056, 100.0867) centre (148.5, 104.9999) ccw projected
  arc A30 (145.4331, 98.9589) -> (145.056, 100.0867) centre (144.482, 99.2679) ccw projected
  line L14 (145.4331, 98.9589) -> (144.1176, 94.9103) projected
  arc A31 (144.1176, 94.9103) -> (146.1149, 94.2614) centre (145.1163, 94.5858) ccw projected
  line L15 (146.1149, 94.2614) -> (147.4303, 98.3099) projected
  arc A32 (148.3983, 99.0008) -> (147.4303, 98.3099) centre (148.3814, 98.0009) ccw projected
  arc A33 (148.3983, 99.0008) -> (148.6017, 99.0008) centre (148.5, 104.9999) ccw projected
  arc A34 (149.5697, 98.3099) -> (148.6017, 99.0008) centre (148.6186, 98.0009) ccw projected
  line L16 (149.5697, 98.3099) -> (150.8851, 94.2614) projected
  arc A35 (150.8851, 94.2614) -> (152.8823, 94.9103) centre (151.8837, 94.5858) ccw projected
  line L17 (152.8823, 94.9103) -> (151.5669, 98.9589) projected
  arc A36 (151.9439, 100.0867) -> (151.5669, 98.9589) centre (152.5179, 99.2679) ccw projected
  arc A37 (151.9439, 100.0867) -> (152.1084, 100.2063) centre (148.5, 104.9999) ccw projected
  arc A38 (153.2976, 100.2163) -> (152.1084, 100.2063) centre (152.7099, 99.4073) ccw projected
  line L18 (153.2976, 100.2163) -> (156.7416, 97.7142) projected
  arc A39 (156.7416, 97.7142) -> (157.9759, 99.4131) centre (157.3587, 98.5637) ccw projected
  line L19 (157.9759, 99.4131) -> (154.532, 101.9153) projected
  arc A40 (154.1741, 103.0494) -> (154.532, 101.9153) centre (155.1198, 102.7243) ccw projected
  point P0 (0, 0)
